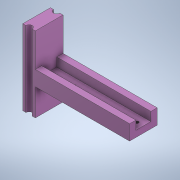
# Autodesk Inventor part: forkmount
Saved by Autodesk Inventor 2022 (Build 260153000, 153)
## iProperties
Created: 2022-11-06
Part Number: forkmount
Material: ABS プラスチック
Document SubType Name: Modeling
Designer: Yazawa
Density: 1.06 g/cm^3
Appearance: 滑らか - 白
Author: Yazawa
Autodesk Inventor part; units mm, degrees
ref_plane "YZ Plane" through (0, 0, 0) normal (1, 0, 0) x (0, 1, 0)
ref_plane "XZ Plane" through (0, 0, 0) normal (0, 1, 0) x (-1, 0, 0)
ref_plane "XY Plane" through (0, 0, 0) normal (0, 0, 1) x (1, 0, 0)
sketch "スケッチ1" plane through (0, 0, 0) normal (0, 1, 0) x (-1, 0, 0)
  line L0 (34, -11) -> (-51, -11)
  line L1 (-51, -11) -> (-51, 11)
  line L2 (-51, 11) -> (34, 11)
  line L3 (34, 11) -> (34, -11)
  line L4 (34, 0) -> (-51, 0) construction
  point P0 (0, 0)
  point P1 (0, 0)
  point P2 (-46, 0)
  dimension "d0" = 22
  dimension "d1" = 85
  dimension "d2" = 5
  dimension "d3" = 46
  constraints: 10 end point, 2 midpoint, 2 parallel, 1 coincident, 1 horizontal, 1 horizontal alignment, 1 perpendicular, 1 point on line
  measures "d0" distance of L2.end L0.start
  measures "d1" distance of L0.start L0.end
  measures "d2" distance from line of point (-46, 0) L1
  measures "d3" distance of point (0, 0) point (-46, 0)
extrude "押し出し1" add sketch "スケッチ1" along normal blind 12
sketch "スケッチ2" plane through (0, 12, 0) normal (0, 1, 0) x (1, 0, 0)
  line L0 (-34, 11) -> (-34, -11) projected
  line L1 (51, -11) -> (51, 11) projected
  line L2 (-34, 0) -> (51, 0)
  line L3 (51, 0) -> (51, 6)
  line L4 (51, 6) -> (-34, 6)
  line L5 (-34, 6) -> (-34, 0)
  line L6 (51, 0) -> (51, -6)
  line L7 (51, -6) -> (-34, -6)
  line L8 (-34, -6) -> (-34, 0)
  point P0 (0, 0)
  point P1 (-34, -6)
  point P2 (-34, 6)
  dimension "d6" = 12
  constraints: 14 end point, 2 parallel, 2 point on line, 2 symmetric about line, 1 horizontal, 1 midpoint, 1 perpendicular
  measures "d6" distance between parallel lines of L7 L4
extrude "押し出し2" cut sketch "スケッチ2" against normal blind 7
sketch "スケッチ3" plane through (0, 5, 0) normal (0, 1, 0) x (1, 0, 0)
  point P0 (0, 0)
  point P1 (-4, 0)
  point P2 (46, 0)
  dimension "d9" = 4
  dimension "d10" = 50
  constraints: 2 horizontal alignment
  measures "d9" distance of point (0, 0) point (-4, 0)
  measures "d10" distance of point (46, 0) point (-4, 0)
hole "穴1" at (-4, 5, 0) at (46, 5, 0) direction (0, -1, 0) diameter 2.459 end through all thread size "M3x0.5" class "6H" standard "ISO Metric profile"
sketch "スケッチ4" plane through (-34, 0, -11) normal (-1, 0, 0) x (0, 0, 1)
  line L0 (0, 38.5) -> (22, 38.5)
  line L1 (22, 38.5) -> (22, -21.5)
  line L2 (22, -21.5) -> (0, -21.5)
  line L3 (0, -21.5) -> (0, 38.5)
  line L4 (0, 0) -> (0, 12) projected
  line L5 (22, 0) -> (22, 12) projected
  line L6 (0, 12) -> (5, 12) construction
  line L7 (5, 12) -> (17, 5) construction
  line L8 (22, 38.5) -> (0, -21.5) construction
  point P0 (11, 0)
  point P1 (11, 8.5)
  dimension "d18" = 60
  constraints: 12 end point, 2 collinear, 2 midpoint, 2 parallel, 1 horizontal, 1 perpendicular
  measures "d18" distance between parallel lines of L0 L2
extrude "押し出し3" add sketch "スケッチ4" against normal blind 10
sketch "スケッチ5" plane through (-34, 38.5, 11) normal (0, 1, 0) x (1, 0, 0)
  line L0 (0, 22) -> (10, 22) projected
  line L1 (0, 0) -> (10, 0) projected
  circle A0 centre (5, 0) radius 2.5
  circle A1 centre (5, 22) radius 2.5
  point P0 (34, 11)
  dimension "d21" = 5
  dimension "d22" = 5
  constraints: 2 centre point, 2 coincident, 2 midpoint
  measures "d21" diameter of A0
  measures "d22" diameter of A1
extrude "押し出し4" cut sketch "スケッチ5" against normal through all
